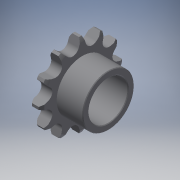
# Autodesk Inventor part: 22252-10380732012
Saved by Autodesk Inventor 2018 (Build 220112000, 112)
## iProperties
Category: PARTsolutions
Company: NORELEM
Created: 2018-08-05
Part Number: 22252-10380732012
Material: Generic
Catalog Web Link: www.cadenas.de
Description: 22252-Sprockets single 3/8“ x 7/32“ DIN ISO 606
Vendor: NORELEM
Document SubType Name: Modeling
Designer: psadmin
Manufacturer: NORELEM
Mass: 13.229 g
Surface Area: 47.6864 cm^2
Volume: 13.229 cm^3
Density: 1 g/cm^3
Appearance: PSOLRGB-175-175-175
PSOL_IDENT_0: {$CADENAS_DATA\23d-libs\norelem\data\22000\22252.prj},174 {VTYP=3D},{NB=22252-10380732012},{LINA=222
PSOL_IDENT_1: 52-10380732012},{NN=22252},{DATE=25.07.2018 05:07:11},{GEOMDATE=17.06.2016 07:26:47},{VERSION=},{LIN
PSOL_IDENT_2: EID=190},{WBVAR=},{WBNUMERIC=}  {NB=22252-10380732012},{LINA=22252-10380732012},{KT=DUMMY},{BEST=222
PSOL_IDENT_3: 52-10380732012},{ISONR=06 B-1},{TZOLL=3/8\" x 7/32\"},{TMM=9,525 x 5,72},{ZZ=12},{D=40.5},{D1=36.80}
PSOL_IDENT_4: ,{D2=25},{D3=8},{B1=5.3},{L=25},{C=1},{R=10},{BS=Infotext},{INFO=Info},{FILTER=NORELEM,},{SAP=212254
PSOL_IDENT_5: },{XC=1.300},{XD=6.350},{XF=1.800},{XG=0.000},{XH=0.000},{XI=0.000},{XJ=0.000},{XK=0.000},{XL=0.000}
PSOL_IDENT_6: ,{XM=0.000},{XN=0.000}
NN: 22252
NT: Sprockets single 3/8“ x 7/32“ DIN ISO 606
NB: 22252-10380732012
NBSYN: $BEST.
LINA: 22252-10380732012
BEST: 22252-10380732012
ISONR: 06 B-1
TZOLL: 3/8" x 7/32"
TMM: 9,525 x 5,72
ZZ: 12
D: 40.5
D1: 36.8
D2: 25
D3: 8
B1: 5.3
L: 25
C: 1
R: 10
BS: Infotext
INFO: Info
SUPPLIER: NORELEM
ARTICLENO: 22252-10380732012
BOMINFO: 22252-10380732012
CREATOR: CADENAS GmbH
Title: 22252-10380732012
Author: Cadenas PARTsolutions
Comments: Sprockets single 3/8“ x 7/32“ DIN ISO 606
Autodesk Inventor part; units mm, degrees
ref_plane "YZ Plane" through (0, 0, 0) normal (1, 0, 0) x (0, 1, 0)
ref_plane "XZ Plane" through (0, 0, 0) normal (0, 1, 0) x (-1, 0, 0)
ref_plane "XY Plane" through (0, 0, 0) normal (0, 0, 1) x (1, 0, 0)
sketch "Sketch_3" plane through (0, 0, 0) normal (1, 0, 0) x (0, 1, 0)
  arc A0 (0, 20.25) -> (-0.65, 20.2396) centre (0, 0) ccw
  line L0 (-0.65, 20.2396) -> (-1.7234, 16.8193)
  arc A1 (-3.9379, 14.6966) -> (-1.7234, 16.8193) centre (-4.7623, 17.773) ccw
  arc A2 (-6.9171, 15.4277) -> (-3.9379, 14.6966) centre (-4.7623, 17.773) ccw
  line L1 (-6.9171, 15.4277) -> (-9.5569, 17.853)
  arc A3 (-9.5569, 17.853) -> (-10.125, 17.537) centre (0, 0) ccw
  arc A4 (-10.125, 17.537) -> (-10.6827, 17.203) centre (0, 0) ccw
  line L2 (-10.6827, 17.203) -> (-9.9022, 13.7042)
  arc A5 (-10.7586, 10.7586) -> (-9.9022, 13.7042) centre (-13.0108, 13.0108) ccw
  arc A6 (-13.7042, 9.9022) -> (-10.7586, 10.7586) centre (-13.0108, 13.0108) ccw
  line L3 (-13.7042, 9.9022) -> (-17.203, 10.6827)
  arc A7 (-17.203, 10.6827) -> (-17.537, 10.125) centre (0, 0) ccw
  arc A8 (-17.537, 10.125) -> (-17.853, 9.5569) centre (0, 0) ccw
  line L4 (-17.853, 9.5569) -> (-15.4277, 6.9171)
  arc A9 (-14.6966, 3.9379) -> (-15.4277, 6.9171) centre (-17.773, 4.7623) ccw
  arc A10 (-16.8193, 1.7234) -> (-14.6966, 3.9379) centre (-17.773, 4.7623) ccw
  line L5 (-16.8193, 1.7234) -> (-20.2396, 0.65)
  arc A11 (-20.2396, 0.65) -> (-20.25, 0) centre (0, 0) ccw
  arc A12 (-20.25, 0) -> (-20.2396, -0.65) centre (0, 0) ccw
  line L6 (-20.2396, -0.65) -> (-16.8193, -1.7234)
  arc A13 (-14.6966, -3.9379) -> (-16.8193, -1.7234) centre (-17.773, -4.7623) ccw
  arc A14 (-15.4277, -6.9171) -> (-14.6966, -3.9379) centre (-17.773, -4.7623) ccw
  line L7 (-15.4277, -6.9171) -> (-17.853, -9.5569)
  arc A15 (-17.853, -9.5569) -> (-17.537, -10.125) centre (0, 0) ccw
  arc A16 (-17.537, -10.125) -> (-17.203, -10.6827) centre (0, 0) ccw
  line L8 (-17.203, -10.6827) -> (-13.7042, -9.9022)
  arc A17 (-10.7586, -10.7586) -> (-13.7042, -9.9022) centre (-13.0108, -13.0108) ccw
  arc A18 (-9.9022, -13.7042) -> (-10.7586, -10.7586) centre (-13.0108, -13.0108) ccw
  line L9 (-9.9022, -13.7042) -> (-10.6827, -17.203)
  arc A19 (-10.6827, -17.203) -> (-10.125, -17.537) centre (0, 0) ccw
  arc A20 (-10.125, -17.537) -> (-9.5569, -17.853) centre (0, 0) ccw
  line L10 (-9.5569, -17.853) -> (-6.9171, -15.4277)
  arc A21 (-3.9379, -14.6966) -> (-6.9171, -15.4277) centre (-4.7623, -17.773) ccw
  arc A22 (-1.7234, -16.8193) -> (-3.9379, -14.6966) centre (-4.7623, -17.773) ccw
  line L11 (-1.7234, -16.8193) -> (-0.65, -20.2396)
  arc A23 (-0.65, -20.2396) -> (0, -20.25) centre (0, 0) ccw
  arc A24 (0, -20.25) -> (0.65, -20.2396) centre (0, 0) ccw
  line L12 (0.65, -20.2396) -> (1.7234, -16.8193)
  arc A25 (3.9379, -14.6966) -> (1.7234, -16.8193) centre (4.7623, -17.773) ccw
  arc A26 (6.9171, -15.4277) -> (3.9379, -14.6966) centre (4.7623, -17.773) ccw
  line L13 (6.9171, -15.4277) -> (9.5569, -17.853)
  arc A27 (9.5569, -17.853) -> (10.125, -17.537) centre (0, 0) ccw
  arc A28 (10.125, -17.537) -> (10.6827, -17.203) centre (0, 0) ccw
  line L14 (10.6827, -17.203) -> (9.9022, -13.7042)
  arc A29 (10.7586, -10.7586) -> (9.9022, -13.7042) centre (13.0108, -13.0108) ccw
  arc A30 (13.7042, -9.9022) -> (10.7586, -10.7586) centre (13.0108, -13.0108) ccw
  line L15 (13.7042, -9.9022) -> (17.203, -10.6827)
  arc A31 (17.203, -10.6827) -> (17.537, -10.125) centre (0, 0) ccw
  arc A32 (17.537, -10.125) -> (17.853, -9.5569) centre (0, 0) ccw
  line L16 (17.853, -9.5569) -> (15.4277, -6.9171)
  arc A33 (14.6966, -3.9379) -> (15.4277, -6.9171) centre (17.773, -4.7623) ccw
  arc A34 (16.8193, -1.7234) -> (14.6966, -3.9379) centre (17.773, -4.7623) ccw
  line L17 (16.8193, -1.7234) -> (20.2396, -0.65)
  arc A35 (20.2396, -0.65) -> (20.25, 0) centre (0, 0) ccw
  arc A36 (20.25, 0) -> (20.2396, 0.65) centre (0, 0) ccw
  line L18 (20.2396, 0.65) -> (16.8193, 1.7234)
  arc A37 (14.6966, 3.9379) -> (16.8193, 1.7234) centre (17.773, 4.7623) ccw
  arc A38 (15.4277, 6.9171) -> (14.6966, 3.9379) centre (17.773, 4.7623) ccw
  line L19 (15.4277, 6.9171) -> (17.853, 9.5569)
  arc A39 (17.853, 9.5569) -> (17.537, 10.125) centre (0, 0) ccw
  arc A40 (17.537, 10.125) -> (17.203, 10.6827) centre (0, 0) ccw
  line L20 (17.203, 10.6827) -> (13.7042, 9.9022)
  arc A41 (10.7586, 10.7586) -> (13.7042, 9.9022) centre (13.0108, 13.0108) ccw
  arc A42 (9.9022, 13.7042) -> (10.7586, 10.7586) centre (13.0108, 13.0108) ccw
  line L21 (9.9022, 13.7042) -> (10.6827, 17.203)
  arc A43 (10.6827, 17.203) -> (10.125, 17.537) centre (0, 0) ccw
  arc A44 (10.125, 17.537) -> (9.5569, 17.853) centre (0, 0) ccw
  line L22 (9.5569, 17.853) -> (6.9171, 15.4277)
  arc A45 (3.9379, 14.6966) -> (6.9171, 15.4277) centre (4.7623, 17.773) ccw
  arc A46 (1.7234, 16.8193) -> (3.9379, 14.6966) centre (4.7623, 17.773) ccw
  line L23 (1.7234, 16.8193) -> (0.65, 20.2396)
  arc A47 (0.65, 20.2396) -> (0, 20.25) centre (0, 0) ccw
  circle A48 centre (0, 0) radius 4
  constraints: 96 point on circle, 49 centre point, 48 end point
extrude "Extrusion1" add sketch "Sketch_3" along normal blind 25
sketch "Sketch_5" plane through (0, 0, 0) normal (0, 0, 1) x (1, 0, 0)
  line L0 (25, 0) -> (-2.65, 0)
  line L1 (-2.65, 25.25) -> (-2.65, 18.45)
  line L2 (-2.65, 18.45) -> (0, 18.45)
  arc A0 (1, 20.25) -> (0, 18.45) centre (9.1951, 14.5194) ccw
  line L3 (1, 20.25) -> (4.3, 20.25)
  arc A1 (5.3, 18.45) -> (4.3, 20.25) centre (-3.8951, 14.5194) ccw
  line L4 (5.3, 18.45) -> (5.3, 12.5)
  line L5 (5.3, 12.5) -> (24.5, 12.5)
  line L6 (24.5, 12.5) -> (25, 12)
  line L7 (25, 12) -> (25, 25.25)
  line L8 (25, 25.25) -> (-2.65, 25.25)
  line L9 (0, 13.7042) -> (25, 13.7042) projected
  line L10 (0, -29.35) -> (0, 34.35) projected
  line L11 (-9.6741, 0) -> (30.779, 0) projected
  dimension "d3" = 3.3
  dimension "d4" = 10
  dimension "d5" = 2.65
  dimension "d6" = 6.8
  dimension "d7" = 27.65
  dimension "d8" = 13.25
  dimension "d9" = 10
  dimension "d10" = 0.5
  dimension "d11" = 0.5
  dimension "d13" = 19.2
  dimension "d14" = 5.95
  dimension "d15" = 7.95
  dimension "d16" = 25.25
  dimension "d17" = 2.65
  dimension "d18" = 5
  dimension "d19" = 1
  dimension "d20" = 1.8
  dimension "d21" = 1.8
  constraints: 18 end point, 4 point on circle, 2 centre point
  measures "d3" distance of L3.start L3.end
  measures "d4" radius of A0
  measures "d5" distance of L1.end L2.end
  measures "d6" distance of L1.start L1.end
  measures "d7" distance of L7.end L1.start
  measures "d8" distance of L6.end L7.end
  measures "d9" radius of A1
  measures "d10" horizontal distance of L5.end L6.end
  measures "d11" distance from line of L7 L5.end
  measures "d13" distance of L4.end L5.end
  measures "d14" distance of L4.start L4.end
  measures "d15" distance between parallel lines of L1 L4
  measures "d16" distance between parallel lines of L11 L8
  measures "d17" distance between parallel lines of L10 L1
  measures "d18" distance between parallel lines of L8 L3
  measures "d19" horizontal distance of L3.end L4.start
  measures "d20" vertical distance of L4.start L3.end
  measures "d21" vertical distance of L3.start L2.end
revolve "Revolution1" cut sketch "Sketch_5" angle 360 about axis through (25, 0, 0) along (1, 0, 0) contours L8 L10 L2 L1 | L8 L7 L9 L4 A1 L3 A0 L10 | L7 L6 L5 L4 L9
sketch "Sketch3" plane through (25, 0, 0) normal (1, 0, 0) x (0, 0, -1)
  circle A0 centre (0, 0) radius 4
  circle A1 centre (0, 0) radius 12.5
  circle A2 centre (0, 0) radius 9.5
  dimension "d24" = 19
  constraints: 3 centre point, 3 coincident
  measures "d24" diameter of A2
extrude "Extrusion2" cut sketch "Sketch3" against normal blind 7 contours A1 | A2
sketch "Sketch4" plane through (0, 0, 0) normal (-1, 0, 0) x (0, 0, 1)
  point P0 (0, 0)
  point P1 (0, 0)
  constraints: 1 coincident
hole "Hole1" at (0, 0, 0) direction (1, 0, 0) diameter 19 end through all
chamfer "Chamfer1" distance 0.3 angle 45 3 edges at (0, 0, -9.5) (18, -12.5, 0) (18, 0, -9.5)
body "Solid1"
